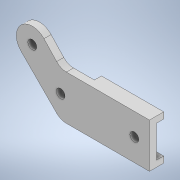
# Autodesk Inventor part: handlesupport
Saved by Autodesk Inventor 2020.3 (Build 243373000, 373)
## iProperties
Created: 2021-06-19
Part Number: handlesupport
Material: Generic
Document SubType Name: Modeling
Designer: 0x6f736f646f
Density: 1 g/cm^3
Appearance: Default
Author: 0x6f736f646f
Autodesk Inventor part; units mm, degrees
ref_plane "YZ Plane" through (0, 0, 0) normal (1, 0, 0) x (0, 1, 0)
ref_plane "XZ Plane" through (0, 0, 0) normal (0, 1, 0) x (-1, 0, 0)
ref_plane "XY Plane" through (0, 0, 0) normal (0, 0, 1) x (1, 0, 0)
sketch "Sketch1" plane through (0, 0, 0) normal (0, 0, 1) x (1, 0, 0)
  line L0 (0, 0) -> (-100, 0)
  line L1 (-100, 0) -> (-100, -50)
  line L2 (-100, -50) -> (0, -50)
  line L3 (0, -50) -> (0, 0)
  line L4 (0, 0) -> (-70, 0)
  line L5 (-70, 0) -> (-70, -50)
  line L6 (-70, -50) -> (0, -50)
  line L7 (0, -50) -> (0, 0)
  line L8 (0, -7) -> (-50, -7)
  line L9 (-50, -7) -> (-50, -43)
  line L10 (-50, -43) -> (0, -43)
  line L11 (0, -43) -> (0, -7)
  line L12 (-100, -24.1908) -> (-131.8198, 7.629)
  line L13 (-100, -24.1908) -> (-55, -24.1908) construction
  circle A0 centre (-131.8198, 7.629) radius 5
  circle A1 centre (-100, -24.1908) radius 5
  circle A2 centre (-17, -25) radius 5
  circle A3 centre (-131.8198, 7.629) radius 18
  line L14 (-100, 0) -> (-118.6863, 19.938)
  line L15 (-100, -50) -> (-144.5979, -5.0486)
  point P0 (0, -43)
  dimension "d0" = 100
  dimension "d1" = 50
  dimension "d2" = 36
  dimension "d3" = 50
  dimension "d4" = 7
  dimension "d5" = 45
  dimension "d6" = 135
  dimension "d7" = 10
  dimension "d8" = 36
  dimension "d9" = 17
  dimension "d10" = 25
  dimension "d11" = 70
  dimension "d13" = 133.144
  constraints: 32 end point, 6 parallel, 4 centre point, 4 horizontal, 3 coincident, 3 perpendicular, 3 point on line, 2 equal radius, 2 point on circle, 2 tangent, 1 equal length
  measures "d0" distance of L1.end L2.end
  measures "d1" distance of L2.end L0.start
  measures "d2" distance between parallel lines of L10 L8
  measures "d3" distance between parallel lines of L3 L9
  measures "d4" distance between parallel lines of L2 L10
  measures "d5" distance of L12.start L12.end
  measures "d6" angle of L13 L12
  measures "d7" diameter of A0
  measures "d8" diameter of A3
  measures "d9" distance from line of L3 A2.centre
  measures "d10" distance from line of L2 A2.centre
  measures "d11" distance between parallel lines of L3 L5
  measures "d13" angle of L0 L14
extrude "Extrusion1" add sketch "Sketch1" along normal blind 8 contours L3 L8 L9 L10 L2 L5 L0 | L5 L2 L1 A1 L0 | L3 L10 L9 L8 | L1 A1 L12 A3 L14 | A3 | L15 A3 L12 A1 L1
extrude "Extrusion2" add sketch "Sketch1" against normal blind 8 contours L3 L8 L9 L10 L2 L5 L0
fillet "Fillet1" radius 15 2 edges at (-100, 0, 4) (-100, -50, 4)
body "Solid1"
